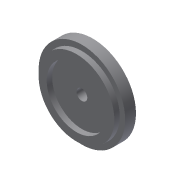
# Autodesk Inventor part: 2sides
Saved by Autodesk Inventor 2022 (Build 260148000, 148)
## iProperties
Shininess: 64.0
Length Units: 11272
Angle Units: 11279
Time Units: 11290
Mass Units: 11286
Length Display Precision: 3
Angle Display Precision: 2
Created: 2002-01-21
Part Number: 2sides
Document SubType Name: Modeling
Designer: Administrator
Density: 1 g/cm^3
Material: Generic
Appearance: Default
Density: 0.0
Volumn: 0.0
Area: 0.0
PropertySet Name: Model Information
Control State: 0
Master: False
Checked Out: False
Author: Administrator
Autodesk Inventor part; units mm, degrees
ref_plane "YZ Plane" through (0, 0, 0) normal (1, 0, 0) x (0, 1, 0)
ref_plane "XZ Plane" through (0, 0, 0) normal (0, 1, 0) x (-1, 0, 0)
ref_plane "XY Plane" through (0, 0, 0) normal (0, 0, 1) x (1, 0, 0)
sketch "Sketch1" plane through (0, 0, 0) normal (0, 0, 1) x (1, 0, 0)
  circle A0 centre (0, 0) radius 25.4
  dimension "d0" = 50.8
  constraints: 1 centre point
  measures "d0" diameter of A0
extrude "Extrusion1" add sketch "Sketch1" along normal blind 6.35
sketch "Sketch2" plane through (0, 0, 6.35) normal (0, 0, 1) x (1, 0, 0)
  circle A0 centre (0, 0) radius 25.4 projected
  circle A1 centre (0, 0) radius 17.4625
  circle A2 centre (0, 0) radius 22.225
  dimension "d3" = 34.925
  dimension "d4" = 44.45
  constraints: 2 centre point, 2 coincident
  measures "d3" diameter of A1
  measures "d4" diameter of A2
extrude "Extrusion2" add sketch "Sketch2" along normal blind 3.175 contours A2
sketch "Sketch3" plane through (0, 0, 0) normal (0, 0, -1) x (-1, 0, 0)
  circle A0 centre (0, 0) radius 25.4 projected
  line L0 (-15.875, 0) -> (-7.9375, 13.7482)
  line L1 (-7.9375, 13.7482) -> (7.9375, 13.7482)
  line L2 (7.9375, 13.7482) -> (15.875, 0)
  line L3 (15.875, 0) -> (7.9375, -13.7482)
  line L4 (7.9375, -13.7482) -> (-7.9375, -13.7482)
  line L5 (-7.9375, -13.7482) -> (-15.875, 0)
  circle A1 centre (0, 0) radius 6.35
  dimension "d7" = 15.875
  dimension "d8" = 12.7
  constraints: 12 end point, 2 coincident, 1 centre point, 11 other
  measures "d7" distance of L3.end L4.end
  measures "d8" diameter of A1
extrude "Extrusion3" add sketch "Sketch3" along normal blind 6.35 contours L0 L1 L2 L3 L4 L5
sketch "Sketch4" plane through (0, 0, 6.35) normal (0, 0, 1) x (1, 0, 0)
  circle A0 centre (0, 0) radius 22.225 projected
  constraints: 1 coincident
hole "Hole1" at (0, 0, 6.35) direction (0, 0, -1) diameter 6.35 end through all
body "Solid1"
